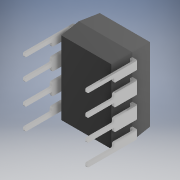
# Autodesk Inventor part: DIP
Saved by Autodesk Inventor 2018 (Build 220112000, 112)
## iProperties
Created: 2017-07-21
Material: Generic
Document SubType Name: Modeling
Designer: Ben
Density: 1 g/cm^3
Appearance: Default
RuleStatus: InUse
Pins: 8.000 ul
Spacing: 2.540 mm
ShoulderWidth: 1.460 mm
PinWidth: 0.450 mm
PackageWidth: 6.350 mm
PackageLength: 9.080 mm
PackageSeatGap: 0.510 mm
PackageHeight: 4.570 mm
PinInsertLength: 3.180 mm
PinThickness: 0.250 mm
PackageAngle: 5.00 deg
PinInsertionSpacing: 7.620 mm
Semi_Circle_Divot: 1.000 ul
Pin_1_Dot: 1.000 ul
Author: Tavan
Autodesk Inventor part; units mm, degrees
sketch "Sketch1" plane through (0, 0, 0) normal (0, 1, 0) x (-1, 0, 0)
  line L0 (-3.175, 4.54) -> (3.175, 4.54)
  line L1 (3.175, 4.54) -> (3.175, -4.54)
  line L2 (3.175, -4.54) -> (-3.175, -4.54)
  line L3 (-3.175, -4.54) -> (-3.175, 4.54)
  line L4 (-3.175, 4.54) -> (3.175, -4.54) construction
  line L5 (3.175, 4.54) -> (-3.175, -4.54) construction
  point P0 (0, 0)
  dimension "d0" = 6.35
  dimension "d1" = 9.08
  constraints: 12 end point, 2 midpoint, 2 parallel, 1 horizontal, 1 perpendicular
  measures "d0" distance of L1.end L2.end
  measures "d1" distance of L0.end L1.end
extrude "Package" add sketch "Sketch1" along normal mid plane 4.57 draft -5
ref_plane "SidePlane1" through (3.175, 0, 0) normal (1, 0, 0) x (0, 1, 0)
ref_plane "SidePlane2" through (-3.175, 0, 0) normal (1, 0, 0) x (0, 1, 0)
ref_plane "EndPlane1" through (0, 0, 4.54) normal (0, 0, 1) x (1, 0, 0)
ref_plane "EndPlane2" through (0, 0, -4.54) normal (0, 0, 1) x (1, 0, 0)
ref_plane "SeatPlane" through (0, -2.795, 0) normal (0, 1, 0) x (-1, 0, 0)
sketch "Sketch2" plane through (0, 0, 4.54) normal (0, 0, 1) x (1, 0, 0)
  line L0 (-3.175, 0) -> (-2.9751, -2.285) projected
  line L1 (-3.175, 0) -> (-3.66, 0)
  line L2 (-3.81, -0.15) -> (-3.81, -0.25)
  line L3 (-3.81, -0.25) -> (-3.56, -0.25) construction
  line L4 (-3.56, -0.4) -> (-3.56, -2.795)
  line L5 (-3.56, -2.795) -> (-3.81, -2.795)
  line L6 (-3.81, -2.795) -> (-3.81, -0.25)
  line L7 (-3.41, -0.25) -> (-3.1531, -0.25)
  arc A0 (-3.66, 0) -> (-3.81, -0.15) centre (-3.66, -0.15) ccw
  arc A1 (-3.41, -0.25) -> (-3.56, -0.4) centre (-3.41, -0.4) ccw
  point P0 (0, 0)
  point P1 (-3.81, 0)
  dimension "d9" = 0.635
  dimension "d10" = 0.25
  dimension "d11" = 0.25
  dimension "d12" = 2.545
  dimension "d13" = 0.15
  constraints: 14 end point, 5 point on line, 4 point on circle, 4 tangent, 3 horizontal, 2 centre point, 2 parallel, 1 equal radius, 1 perpendicular, 1 vertical
  measures "d9" distance of L0.start point (-3.81, 0)
  measures "d10" distance of point (-3.81, 0) L2.end
  measures "d11" distance of L4.end L5.end
  measures "d12" distance of L3.end L4.end
  measures "d13" radius of A0
extrude "Shoulder" add sketch "Sketch2" against normal blind 1.46 separate body
sketch "Sketch3" plane through (-3.81, -2.795, 4.54) normal (0, -1, 0) x (1, 0, 0)
  line L0 (0.25, -1.46) -> (0, -1.46) projected
  line L1 (0, 0) -> (0, -1.46) projected
  line L2 (0, 0) -> (0, -1.46) construction
  line L3 (0, -0.73) -> (0.125, -0.73) construction
  line L4 (0.25, -0.505) -> (0, -0.505)
  line L5 (0, -0.505) -> (0, -0.955)
  line L6 (0, -0.955) -> (0.25, -0.955)
  line L7 (0.25, -0.955) -> (0.25, -0.505)
  line L8 (0.25, -0.505) -> (0, -0.955) construction
  line L9 (0, -0.505) -> (0.25, -0.955) construction
  point P0 (3.81, -4.54)
  dimension "d16" = 0.25
  dimension "d17" = 0.45
  constraints: 14 end point, 3 midpoint, 2 horizontal, 2 parallel, 1 perpendicular
  measures "d16" distance of L6.end L5.end
  measures "d17" distance of L5.end L4.end
extrude "Insertion" add sketch "Sketch3" along normal blind 3.18 bodies 2
fillet "PinFillet" radius 0.15 6 edges at (-3.685, -2.795, 3.08) (-3.685, -2.795, 4.54) (-3.685, -2.795, 4.035) (-3.685, -2.795, 3.585) (-3.685, -5.975, 3.585) (-3.685, -5.975, 4.035)
pattern_linear "PinLine" count 4 spacing 2.54 along (0, 0, -1) of "Shoulder", "Insertion", "PinFillet" bodies 2
mirror "DualLine" about plane through (0, 0, 0) normal (1, 0, 0) of "Shoulder", "Insertion", "PinFillet", "PinLine" bodies 2
sketch "Sketch4" plane through (0, 0, 4.54) normal (0, 0, 1) x (1, 0, 0)
  line L0 (4.5, 4.5) -> (-4.5, 4.5)
  line L1 (-4.5, 4.5) -> (-4.5, -4.5)
  line L2 (-4.5, -4.5) -> (4.5, -4.5)
  line L3 (4.5, -4.5) -> (4.5, 4.5)
  line L4 (3.175, 0) -> (-3.175, 0) projected
  line L5 (4.5, 4.5) -> (-4.5, -4.5) construction
  line L6 (-4.5, 4.5) -> (4.5, -4.5) construction
  point P0 (0, 0)
  dimension "d26" = 9
  dimension "d27" = 9
  constraints: 12 end point, 3 midpoint, 2 parallel, 1 horizontal, 1 perpendicular
  measures "d26" distance of L2.end L1.end
  measures "d27" distance of L1.end L0.end
extrude "EdgePinCut1" cut sketch "Sketch4" against normal blind 0.505 bodies 2
sketch "Sketch5" plane through (0, 0, -4.54) normal (0, 0, 1) x (1, 0, 0)
  line L0 (-4.5, 4.5) -> (4.5, 4.5)
  line L1 (4.5, 4.5) -> (4.5, -4.5)
  line L2 (4.5, -4.5) -> (-4.5, -4.5)
  line L3 (-4.5, -4.5) -> (-4.5, 4.5)
  line L4 (-4.5, 4.5) -> (4.5, -4.5) construction
  line L5 (4.5, 4.5) -> (-4.5, -4.5) construction
  point P0 (0, 0)
  dimension "d30" = 9
  dimension "d31" = 9
  constraints: 12 end point, 2 midpoint, 2 parallel, 1 horizontal, 1 perpendicular
  measures "d30" distance of L1.end L2.end
  measures "d31" distance of L0.end L1.end
extrude "EdgePinCut2" cut sketch "Sketch5" along normal blind 0.505 bodies 2
sketch "Sketch6" plane through (0, 2.285, 0) normal (0, 1, 0) x (1, 0, 0)
  line L0 (-3.175, 4.54) -> (3.175, 4.54) projected
  arc A0 (-1, 4.54) -> (1, 4.54) centre (0, 4.54) ccw
  point P0 (0, 0)
  dimension "d34" = 1
  constraints: 2 point on circle, 2 point on line, 1 centre point, 1 midpoint
  measures "d34" radius of A0
extrude "SemiCircleDivot" cut sketch "Sketch6" against normal blind 0.5 bodies 1
sketch "Sketch7" plane through (0, 2.285, 0) normal (0, 1, 0) x (1, 0, 0)
  line L0 (-2.9751, 4.3401) -> (2.9751, 4.3401) projected
  line L1 (-2.9751, -4.3401) -> (-2.9751, 4.3401) projected
  circle A0 centre (-2.4751, 3.8401) radius 0.25
  point P0 (0, 0)
  point P1 (-0.9798, 4.3401)
  dimension "d37" = 0.5
  dimension "d38" = 0.5
  dimension "d39" = 0.5
  constraints: 1 centre point
  measures "d37" diameter of A0
  measures "d38" distance from line of L0 A0.centre
  measures "d39" distance from line of L1 A0.centre
extrude "Pin1Dot" cut sketch "Sketch7" against normal blind 0.01 bodies 1
equation "\"d0\" = PackageWidth"
equation "\"d1\" = PackageLength"
equation "\"d2\" = PackageHeight"
equation "\"d3\" = -PackageAngle"
equation "\"d9\" = -0.5 * PackageWidth + 0.5 * PinInsertionSpacing"
equation "\"d10\" = PinThickness"
equation "\"d11\" = PinThickness"
equation "\"d12\" = PackageSeatGap + 0.5 * PackageHeight - PinThickness"
equation "\"d14\" = ShoulderWidth"
equation "\"d16\" = PinThickness"
equation "\"d17\" = PinWidth"
equation "\"d18\" = PinInsertLength"
equation "\"d23\" = Spacing"
equation "\"d28\" = 0.5 * ShoulderWidth - 0.5 * PinWidth"
equation "\"d32\" = 0.5 * ShoulderWidth - 0.5 * PinWidth"
equation "\"Spacing\" = 2.54"
equation "\"ShoulderWidth\" = 1.46"
equation "\"PinWidth\" = 0.45"
equation "\"PackageWidth\" = 6.35"
equation "\"PackageLength\" = 9.08"
equation "\"PackageHeightFromSeat\" = 5.08"
equation "\"PackageSeatGap\" = 0.51"
equation "\"PackageHeight\" = PackageHeightFromSeat - PackageSeatGap"
equation "\"PinInsertLength\" = 3.18"
equation "\"GaugePlane\" = 0.38"
equation "\"PinThickness\" = 0.25"
equation "\"PackageAngle\" = 5deg"
equation "\"d4\" = 0.5 * PackageWidth"
equation "\"d5\" = 0.5 * PackageLength"
equation "\"d7\" = -0.5 * PackageLength"
equation "\"d8\" = -0.5 * PackageWidth"
equation "\"PinInsertionSpacing\" = 7.62"
equation "\"d42\" = -PackageHeightFromSeat + 0.5 * PackageHeight"
body "Solid1"
body "Solid2"
